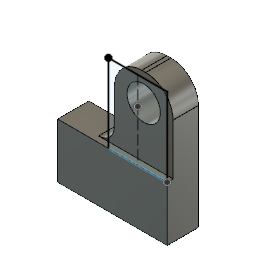
throttle bracket v3 (Autodesk Fusion 360 design; units mm, degrees)
Autodesk Fusion 360 part; units mm, degrees
box "BoxPrimitive1" add length 8 width 28 height 14 placed x (0, 0, 1) y (1, 0, 0) z (0, 1, 0) at (-28, 0, 0)
box "BoxPrimitive2" add length 8 width 15 height 20 placed x (0, 0, 1) y (1, 0, 0) z (0, 1, 0) at (-15, 14, 0)
sketch "Sketch4" plane through (0, 0, 8) normal (0, 0, 1) x (1, 0, 0)
  line L0 (-28, 14) -> (-28, 0)
  line L1 (-28, 0) -> (0, 0)
  line L2 (0, 0) -> (0, 34)
  line L3 (0, 34) -> (-15, 34)
  line L4 (-15, 34) -> (-15, 14)
  line L5 (-15, 14) -> (-28, 14)
  line L6 (-15, 34) -> (0, 34)
  line L7 (0, 34) -> (0, 14)
  line L8 (0, 14) -> (-15, 14)
  line L9 (-15, 14) -> (-15, 34)
  line L10 (-7.5, 34) -> (-7.5, 14) construction
  point P0 (-7.5, 27)
  dimension "holeHeight" = 13
  constraint horizontal L6
  constraint vertical L7
  constraint horizontal L8
  constraint vertical L9
  constraint coincident L2 L7.end
  constraint coincident L3.end L4.start
  constraint midpoint L3 L10.start
  constraint midpoint L8 L10.end
  constraint coincident L10 P0
  measures "holeHeight" distance of L10.end P0
hole "Hole1" at (-7.5, 27, 8) direction (0, 0, -1) diameter 8.5 end through all
extrude "Extrude1" cut sketch "Sketch4" against normal blind 1.5 contours L2 L3 L4 L6 L7 L8 L9
fillet "Fillet2" radius 7 2 edges at (-15, 34, 3.25) (0, 34, 3.25)
fillet "Fillet3" radius 4 1 edges at (-15, 14, 3.25)
